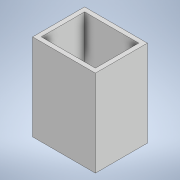
# Autodesk Inventor part: axis_rf+fix
Saved by Autodesk Inventor 2022 (Build 260153000, 153)
## iProperties
Created: 2023-03-23
Part Number: axis_rf+fix
Material: 一般
Document SubType Name: Modeling
Designer: JOU
Density: 1 g/cm^3
Appearance: 預設
Author: JOU
Autodesk Inventor part; units mm, degrees
ref_plane "YZ Plane" through (0, 0, 0) normal (1, 0, 0) x (0, 1, 0)
ref_plane "XZ Plane" through (0, 0, 0) normal (0, 1, 0) x (-1, 0, 0)
ref_plane "XY Plane" through (0, 0, 0) normal (0, 0, 1) x (1, 0, 0)
sketch "草圖1" plane through (0, 0, 0) normal (0, 1, 0) x (-1, 0, 0)
  line L0 (4.4578, 4.5382) -> (-8.0422, 4.5382)
  line L1 (-8.0422, 4.5382) -> (-8.0422, -5.4618)
  line L2 (-8.0422, -5.4618) -> (4.4578, -5.4618)
  line L3 (4.4578, -5.4618) -> (4.4578, 4.5382)
  line L4 (5.4578, -6.4618) -> (-9.0422, -6.4618)
  line L5 (-9.0422, -6.4618) -> (-9.0422, 5.5382)
  line L6 (-9.0422, 5.5382) -> (5.4578, 5.5382)
  line L7 (5.4578, 5.5382) -> (5.4578, -6.4618)
  point P0 (0, 0)
  dimension "d0" = 10
  dimension "d1" = 12.5
  dimension "d2" = 1
  constraints: 16 end point, 4 parallel, 2 perpendicular, 1 horizontal, 3 other
  measures "d0" distance of L2.end L0.start
  measures "d1" distance of L1.end L2.end
  measures "d2" distance between parallel lines of L2 L4
extrude "擠出1" add sketch "草圖1" along normal blind 20
